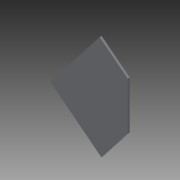
# Autodesk Inventor part: side plate
Saved by Autodesk Inventor 2015 (Build 190159000, 159)
## iProperties
Created: 2015-02-06
Part Number: side plate
Material: Generic
Document SubType Name: Modeling
Designer: degan
Density: 1 g/cm^3
Appearance: Default
Author: degan
Autodesk Inventor part; units mm, degrees
ref_plane "YZ Plane" through (0, 0, 0) normal (1, 0, 0) x (0, 1, 0)
ref_plane "XZ Plane" through (0, 0, 0) normal (0, 1, 0) x (-1, 0, 0)
ref_plane "XY Plane" through (0, 0, 0) normal (0, 0, 1) x (1, 0, 0)
ref_plane "Work Plane1" through (0, 0, 0) normal (0, 0, 1) x (1, 0, 0)
sketch "Sketch1" plane through (0, 0, 0) normal (0, 0, 1) x (1, 0, 0)
  line L0 (-44.45, -52.3787) -> (-44.45, 0) projected
  line L1 (-54.0657, 7.5126) -> (-44.45, 0) projected
  line L2 (-54.0657, 7.5126) -> (-147.8925, -112.5803) projected
  line L3 (-112.8654, -139.9464) -> (-147.8925, -112.5803) projected
  line L4 (-44.45, -52.3787) -> (-112.8654, -139.9464) projected
  line L5 (-121.3082, -78.554) -> (-41.2463, -141.1052)
  line L6 (-41.2463, -141.1052) -> (0, -88.3123)
  line L7 (-121.3082, -78.554) -> (-43.959, 20.4484)
  line L8 (-43.959, 20.4484) -> (0, -13.8961)
  line L9 (-44.45, -203.2) -> (-44.45, 0)
  line L10 (-44.45, 0) -> (0, 0)
  line L11 (0, 0) -> (0, -203.2)
  line L12 (0, -203.2) -> (-44.45, -203.2)
  line L13 (0, -13.8961) -> (0, -88.3123)
  dimension "d0" = 101.6
  dimension "d1" = 43.18
  constraints: 18 end point, 3 perpendicular, 3 point on line, 2 horizontal, 2 vertical, 2 other
  measures "d0" distance of L5.start L5.end
  measures "d1" distance of L2.end L5.start
extrude "Extrusion1" add sketch "Sketch1" along normal blind 3.175 contours L4 L5 L2 L1 L0 | L9 L5 L4 | L0 L10 L8 L11 L6 L5 L9 | L1 L7 L8 L10
body "Solid1"
